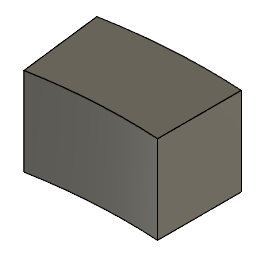
OpenATC-Shock-absorber (Autodesk Fusion 360 design; units mm, degrees)
Autodesk Fusion 360 part; units mm, degrees
sketch "Sketch1" plane through (0, 0, 0) normal (0, 0, 1) x (1, 0, 0)
  line L0 (0, 0) -> (-9.0099, 73.3797)
  line L1 (0, 0) -> (0, 8.9683)
  line L2 (0, 8.9683) -> (0, 73.9307)
  line L3 (-9.0099, 73.3797) -> (-9.7404, 79.3294)
  line L4 (0, 73.9307) -> (0, 79.9251)
  arc A0 (0, 73.9307) -> (-9.0099, 73.3797) centre (-2.263, 37) ccw
  arc A1 (0, 79.9251) -> (-9.7404, 79.3294) centre (-2.4465, 40) ccw
  line L5 (0, 0) -> (0, 2.8792)
  line L6 (0, 0) -> (-8.5021, 139.0084) construction
  dimension "d1" = 37
  dimension "d2" = 40
  dimension "d4" = 3.5
  dimension "d5" = 37
  dimension "d6" = 40
  dimension "d7" = 3.5
  constraint coincident L0.start L1.start
  constraint vertical L1
  constraint parallel L1 L2
  constraint parallel L0 L3
  constraint parallel L2 L4
  constraint coincident L1 L5.end
  constraint coincident A1.centre L6
  constraint coincident A0.centre L6
  measures "d1" radius of A0
  measures "d2" radius of A1
  measures "d4" angle of L4 L6
  measures "d5" vertical distance of L0.start A0.centre
  measures "d6" vertical distance of L0.start A1.centre
  measures "d7" angle of L0 L6
extrude "Extrude1" add sketch "Sketch1" along normal blind 6.3 contours L3 L4 A0 A1
equation "d5 = d1"
equation "d6 = d2"
equation "d7 = d4"
